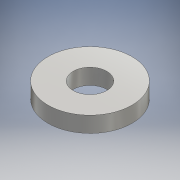
# Autodesk Inventor part: ステンレスワッシャー　t1.5　8-3.2
Saved by Autodesk Inventor 2016 (Build 200138000, 138)
## iProperties
Created: 2018-03-28
Part Number: ステンレスワッシャー　t1.5　8-3.2
Material: ステンレス鋼 AISI 304
Document SubType Name: Modeling
Designer: Takumi
Density: 8 g/cm^3
Appearance: クローム - サテン
Mass: 0.506676 g
Surface Area: 1.37225 cm^2
Volume: 0.0633345 cm^3
Author: Takumi
Autodesk Inventor part; units mm, degrees
ref_plane "YZ Plane" through (0, 0, 0) normal (1, 0, 0) x (0, 1, 0)
ref_plane "XZ Plane" through (0, 0, 0) normal (0, 1, 0) x (-1, 0, 0)
ref_plane "XY Plane" through (0, 0, 0) normal (0, 0, 1) x (1, 0, 0)
sketch "スケッチ1" plane through (0, 0, 0) normal (0, 0, 1) x (1, 0, 0)
  circle A0 centre (0, 0) radius 1.6
  circle A1 centre (0, 0) radius 4
  dimension "d0" = 3.2
  dimension "d1" = 8
  constraints: 2 centre point, 2 coincident
  measures "d0" diameter of A0
  measures "d1" diameter of A1
extrude "押し出し1" add sketch "スケッチ1" along normal blind 1.5
